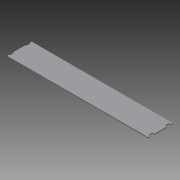
# Autodesk Inventor part: Wing
Saved by Autodesk Inventor 2013 (Build 170138000, 138)
## iProperties
Created: 2013-01-27
Part Number: Wing
Material: Generic
Document SubType Name: Modeling
Designer: Andrew Toennies
Density: 1 g/cm^3
Mass: 115.222 g
Surface Area: 759.878 cm^2
Volume: 115.222 cm^3
Author: Andrew Toennies
Autodesk Inventor part; units mm, degrees
ref_plane "YZ Plane" through (0, 0, 0) normal (1, 0, 0) x (0, 1, 0)
ref_plane "XZ Plane" through (0, 0, 0) normal (0, 1, 0) x (-1, 0, 0)
ref_plane "XY Plane" through (0, 0, 0) normal (0, 0, 1) x (1, 0, 0)
sketch "Sketch1" plane through (0, 0, 0) normal (0, 1, 0) x (-1, 0, 0)
  line L0 (0, 0) -> (558.8, 0)
  line L1 (558.8, 0) -> (558.8, 79.375)
  line L2 (558.8, 79.375) -> (0, 79.375)
  line L3 (0, 79.375) -> (0, 0)
  dimension "d0" = 79.375
  dimension "d1" = 558.8
  constraints: 8 end point, 2 parallel, 1 horizontal, 1 perpendicular
  measures "d0" distance of L2.end L0.start
  measures "d1" distance of L1.end L2.end
extrude "Extrusion1" add sketch "Sketch1" along normal blind 3.175
sketch "Sketch3" plane through (-558.8, 0, 0) normal (-1, 0, 0) x (0, 0, 1)
  line L0 (0, 0) -> (79.375, 0) projected
  line L1 (79.375, 0) -> (79.375, 3.175) projected
  line L2 (0, 3.175) -> (79.375, 3.175) projected
  line L3 (0, 0) -> (0, 3.175) projected
  line L4 (73.025, 3.175) -> (73.025, 0)
  line L5 (60.325, 0) -> (60.325, 3.175)
  line L6 (19.05, 0) -> (19.05, 3.175)
  line L7 (6.35, 0) -> (6.35, 3.175)
  dimension "d4" = 12.7
  dimension "d5" = 6.35
  dimension "d6" = 12.7
  dimension "d7" = 6.35
  constraints: 8 end point, 8 point on line, 4 perpendicular
  measures "d4" distance between parallel lines of L5 L4
  measures "d5" distance between parallel lines of L1 L4
  measures "d6" distance between parallel lines of L6 L7
  measures "d7" distance between parallel lines of L3 L7
extrude "Extrusion2" cut sketch "Sketch3" against normal blind 3.175 contours L7 L2 L6 L0 | L5 L2 L4 L0
sketch "Sketch4" plane through (0, 0, 79.375) normal (1, 0, 0) x (0, 0, -1)
  line L0 (19.05, 3.175) -> (6.35, 3.175) projected
  line L1 (19.05, 0) -> (19.05, 3.175) projected
  line L2 (6.35, 0) -> (19.05, 0) projected
  line L3 (6.35, 3.175) -> (6.35, 0) projected
  line L4 (60.325, 3.175) -> (60.325, 0) projected
  line L5 (73.025, 3.175) -> (60.325, 3.175) projected
  line L6 (73.025, 0) -> (73.025, 3.175) projected
  line L7 (60.325, 0) -> (73.025, 0) projected
extrude "Extrusion3" cut sketch "Sketch4" against normal blind 6.35
body "Solid1"
